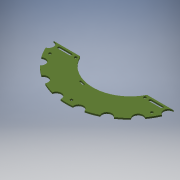
# Autodesk Inventor part: Board_Shape
Saved by Autodesk Inventor 2016 (Build 200138000, 138)
## iProperties
Created: 2015-08-05
Part Number: Board_Shape
Material: Generic
Document SubType Name: Modeling
Designer: 3DPrinterUser
Density: 1 g/cm^3
Appearance: Olive Green
Author: 3DPrinterUser
Autodesk Inventor part; units mm, degrees
ref_plane "YZ Plane" through (0, 0, 0) normal (1, 0, 0) x (0, 1, 0)
ref_plane "XZ Plane" through (0, 0, 0) normal (0, 1, 0) x (-1, 0, 0)
ref_plane "XY Plane" through (0, 0, 0) normal (0, 0, 1) x (1, 0, 0)
sketch "Sketch1" plane through (0, 0, 0) normal (0, 0, 1) x (1, 0, 0)
  circle A0 centre (46.9447, 34.7427) radius 1.05 projected
  circle A1 centre (53.4135, 34.1066) radius 1.05 projected
  circle A2 centre (-46.9447, -34.7427) radius 1.05 construction
  circle A3 centre (-53.4135, -34.1066) radius 1.05 construction
  arc A4 (72.8675, -20.1416) -> (68.7665, -31.409) centre (71.0408, -25.8567) ccw projected
  arc A5 (72.8675, -20.1416) -> (72.8675, 20.1416) centre (0, 0) ccw projected
  arc A6 (68.7665, 31.409) -> (72.8675, 20.1416) centre (71.0408, 25.8567) ccw projected
  arc A7 (68.7665, 31.409) -> (61.5843, 43.8491) centre (0, 0) ccw projected
  arc A8 (53.8769, 53.0343) -> (61.5843, 43.8491) centre (57.913, 48.5947) ccw projected
  arc A9 (53.8769, 53.0343) -> (42.873, 62.2677) centre (0, 0) ccw projected
  arc A10 (32.4889, 68.263) -> (42.873, 62.2677) centre (37.8, 65.4715) ccw projected
  arc A11 (32.4889, 68.263) -> (18.9906, 73.1759) centre (0, 0) ccw projected
  arc A12 (7.1823, 75.2581) -> (18.9906, 73.1759) centre (13.1278, 74.4515) ccw projected
  arc A13 (7.1823, 75.2581) -> (-7.1823, 75.2581) centre (0, 0) ccw projected
  arc A14 (-18.9906, 73.1759) -> (-7.1823, 75.2581) centre (-13.1278, 74.4515) ccw projected
  arc A15 (-18.9906, 73.1759) -> (-32.4889, 68.263) centre (0, 0) ccw projected
  arc A16 (-42.873, 62.2677) -> (-32.4889, 68.263) centre (-37.8, 65.4715) ccw projected
  arc A17 (-42.873, 62.2677) -> (-53.8769, 53.0343) centre (0, 0) ccw projected
  arc A18 (-61.5843, 43.8491) -> (-53.8769, 53.0343) centre (-57.913, 48.5947) ccw projected
  arc A19 (-61.5843, 43.8491) -> (-68.7665, 31.409) centre (0, 0) ccw projected
  arc A20 (-72.8675, 20.1416) -> (-68.7665, 31.409) centre (-71.0408, 25.8567) ccw projected
  arc A21 (-72.8675, 20.1416) -> (-72.8675, -20.1416) centre (0, 0) ccw projected
  arc A22 (-68.7665, -31.409) -> (-72.8675, -20.1416) centre (-71.0408, -25.8567) ccw projected
  arc A23 (-68.7665, -31.409) -> (-61.5843, -43.8491) centre (0, 0) ccw projected
  arc A24 (-53.8769, -53.0343) -> (-61.5843, -43.8491) centre (-57.913, -48.5947) ccw projected
  arc A25 (-53.8769, -53.0343) -> (-42.873, -62.2677) centre (0, 0) ccw projected
  arc A26 (-32.4889, -68.263) -> (-42.873, -62.2677) centre (-37.8, -65.4715) ccw projected
  arc A27 (-32.4889, -68.263) -> (-18.9906, -73.1759) centre (0, 0) ccw projected
  arc A28 (-7.1823, -75.2581) -> (-18.9906, -73.1759) centre (-13.1278, -74.4515) ccw projected
  arc A29 (-7.1823, -75.2581) -> (7.1823, -75.2581) centre (0, 0) ccw projected
  arc A30 (18.9906, -73.1759) -> (7.1823, -75.2581) centre (13.1278, -74.4515) ccw projected
  arc A31 (18.9906, -73.1759) -> (32.4889, -68.263) centre (0, 0) ccw projected
  arc A32 (42.873, -62.2677) -> (32.4889, -68.263) centre (37.8, -65.4715) ccw projected
  arc A33 (42.873, -62.2677) -> (53.8769, -53.0343) centre (0, 0) ccw projected
  arc A34 (61.5843, -43.8491) -> (53.8769, -53.0343) centre (57.913, -48.5947) ccw projected
  arc A35 (61.5843, -43.8491) -> (68.7665, -31.409) centre (0, 0) ccw projected
  circle A36 centre (0, 0) radius 44.3 projected
  circle A37 centre (-69.95, -11.5) radius 1.3 projected
  circle A38 centre (-46.95, 11.5) radius 1.3 projected
  circle A39 centre (69.95, -11.5) radius 1.3 projected
  circle A40 centre (46.95, 11.5) radius 1.3 projected
  circle A41 centre (69.95, 11.5) radius 1.3 projected
  circle A42 centre (46.95, -11.5) radius 1.3 projected
  circle A43 centre (-69.95, 11.5) radius 1.3 projected
  circle A44 centre (-46.95, -11.5) radius 1.3 projected
  circle A45 centre (-58.45, 0) radius 11.5 projected
  circle A46 centre (58.45, 0) radius 11.5 projected
  circle A47 centre (60.2754, -34.8) radius 1.55 projected
  circle A48 centre (44.738, -53.3167) radius 1.55 projected
  circle A49 centre (16.1776, -44.4475) radius 1.55 projected
  circle A50 centre (0, -69.6) radius 1.55 projected
  circle A51 centre (-23.8046, -65.4026) radius 1.55 projected
  circle A52 centre (-30.4039, -36.2339) radius 1.55 projected
  circle A53 centre (-60.2754, -34.8) radius 1.55 projected
  circle A54 centre (60.2754, 34.8) radius 1.55 projected
  circle A55 centre (44.738, 53.3167) radius 1.55 projected
  circle A56 centre (23.8046, 65.4026) radius 1.55 projected
  circle A57 centre (-40.963, 23.65) radius 1.55 projected
  circle A58 centre (-30.4039, 36.2339) radius 1.55 projected
  circle A59 centre (-16.1776, 44.4475) radius 1.55 projected
  circle A60 centre (0, 47.3) radius 1.55 projected
  circle A61 centre (0, 69.6) radius 1.55 projected
  circle A62 centre (-23.8046, 65.4026) radius 1.55 projected
  circle A63 centre (-44.738, 53.3167) radius 1.55 projected
  circle A64 centre (-60.2754, 34.8) radius 1.55 projected
  circle A65 centre (16.1776, 44.4475) radius 1.55 projected
  circle A66 centre (30.4039, 36.2339) radius 1.55 projected
  circle A67 centre (40.963, 23.65) radius 1.55 projected
  circle A68 centre (-40.963, -23.65) radius 1.55 projected
  circle A69 centre (-44.738, -53.3167) radius 1.55 projected
  circle A70 centre (-16.1776, -44.4475) radius 1.55 projected
  circle A71 centre (0, -47.3) radius 1.55 projected
  circle A72 centre (23.8046, -65.4026) radius 1.55 projected
  circle A73 centre (30.4039, -36.2339) radius 1.55 projected
  circle A74 centre (40.963, -23.65) radius 1.55 projected
  line L0 (58.45, 0) -> (0, 0) construction
  line L1 (71.0408, -19.8567) -> (39.6005, -19.8567)
  line L2 (-71.0408, -19.8567) -> (-39.6005, -19.8567)
  point P0 (0, 0)
  constraints: 6 end point, 4 point on circle, 2 tangent, 1 collinear, 1 horizontal, 1 parallel
extrude "Extrusion1" add sketch "Sketch1" along normal blind 1.75 contours A4 A35 A34 A33 A32 A31 A30 A29 A28 A27 A26 A25 A24 A23 A22 L2 A36 L1
sketch "Sketch2" plane through (0, 0, 1.75) normal (0, 0, 1) x (1, 0, 0)
  circle A0 centre (-30.4039, -36.2339) radius 1.55 projected
  circle A1 centre (-44.738, -53.3167) radius 1.55 projected
  circle A2 centre (-23.8046, -65.4026) radius 1.55 projected
  circle A3 centre (-16.1776, -44.4475) radius 1.55 projected
  circle A4 centre (16.1776, -44.4475) radius 1.55 projected
  circle A5 centre (23.8046, -65.4026) radius 1.55 projected
  circle A6 centre (44.738, -53.3167) radius 1.55 projected
  circle A7 centre (30.4039, -36.2339) radius 1.55 projected
  circle A8 centre (0, -47.3) radius 1.55 projected
  point P0 (0, 0)
extrude "Extrusion2" add sketch "Sketch2" against normal up to surface (1.75 mm away)
sketch "Sketch3" plane through (0, 0, 1.75) normal (0, 0, 1) x (1, 0, 0)
  line L0 (-60.9095, -23.5192) -> (-47.1128, -23.5192) construction
  line L1 (-60.9095, -25.0192) -> (-47.1128, -25.0192)
  line L2 (-47.1128, -22.0192) -> (-60.9095, -22.0192)
  arc A0 (-60.9095, -22.0192) -> (-60.9095, -25.0192) centre (-60.9095, -23.5192) ccw
  arc A1 (-47.1128, -25.0192) -> (-47.1128, -22.0192) centre (-47.1128, -23.5192) ccw
  line L3 (-60.9095, -23.5192) -> (-65.5148, -23.5192) construction
  arc A2 (-68.7665, -31.409) -> (-71.0408, -19.8567) centre (-71.0408, -25.8567) ccw projected
  line L4 (-47.1128, -23.5192) -> (-42.5075, -23.5192) construction
  circle A3 centre (-40.963, -23.65) radius 1.55 projected
  point P0 (0, 0)
  point P1 (-54.0112, -23.5192)
  dimension "d4" = 3
  constraints: 12 end point, 5 point on circle, 4 tangent, 2 centre point, 2 horizontal, 1 collinear, 1 midpoint, 1 parallel, 1 point on line, 2 other
  measures "d4" diameter of A1
extrude "Extrusion3" cut sketch "Sketch3" against normal up to surface (1.75 mm away) contours A0 L2 A1 L1
mirror "Mirror1" about plane through (0, 0, 0) normal (1, 0, 0) of "Extrusion3"
sketch "Sketch4" plane through (0, 0, 1.75) normal (0, 0, 1) x (1, 0, 0)
  line L0 (-13.6091, -45.3689) -> (-8.7507, -46.5507) construction
  line L1 (-13.8454, -46.3405) -> (-8.9871, -47.5223)
  line L2 (-8.5144, -45.579) -> (-13.3727, -44.3972)
  arc A0 (-13.3727, -44.3972) -> (-13.8454, -46.3405) centre (-13.6091, -45.3689) ccw
  arc A1 (-8.9871, -47.5223) -> (-8.5144, -45.579) centre (-8.7507, -46.5507) ccw
  circle A2 centre (0, 0) radius 47.3 construction
  arc A3 (-39.6005, -19.8567) -> (39.6005, -19.8567) centre (0, 0) ccw projected
  point P0 (-11.1799, -45.9598)
  dimension "d7" = 2
  dimension "d8" = 5
  dimension "d9" = 2
  constraints: 8 end point, 4 point on circle, 4 tangent, 2 centre point, 1 coincident, 1 midpoint, 1 parallel, 4 other
  measures "d7" diameter of A1
  measures "d8" distance of L0.start L0.end
  measures "d9" distance edge to line of A3 L2
extrude "Extrusion4" cut sketch "Sketch4" against normal up to surface (1.75 mm away)
equation "\"d0\" = board_height"
equation "\"d2\" = board_height"
equation "\"d5\" = board_height"
equation "\"d10\" = board_height"
equation "\"board_height\" = 1.75"
body "Solid1"
